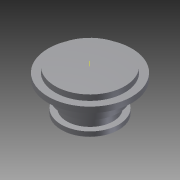
# Autodesk Inventor part: GL45 bottle cap insert; solid
Saved by Autodesk Inventor 2011 (Build 150239000, 239)
## iProperties
Created: 2012-03-14
Part Number: GL45 bottle cap insert; solid
Document SubType Name: Modeling
Designer: Marc
Density: 1 g/cm^3
Author: Marc
Autodesk Inventor part; units mm, degrees
ref_plane "YZ Plane" through (0, 0, 0) normal (1, 0, 0) x (0, 1, 0)
ref_plane "XZ Plane" through (0, 0, 0) normal (0, 1, 0) x (-1, 0, 0)
ref_plane "XY Plane" through (0, 0, 0) normal (0, 0, 1) x (1, 0, 0)
sketch "Sketch1" plane through (0, 0, 0) normal (0, 0, 1) x (1, 0, 0)
  line L0 (0, 0) -> (-14.478, 0)
  line L1 (-14.478, 0) -> (-14.478, 2.54)
  line L2 (-14.478, 2.54) -> (-11.684, 2.54)
  line L3 (-11.684, 2.54) -> (-11.684, 7.62)
  line L4 (-11.684, 7.62) -> (-14.478, 7.62)
  line L5 (-14.478, 7.62) -> (-14.478, 15.24)
  line L6 (-14.478, 15.24) -> (-21.082, 15.24)
  line L7 (-21.082, 15.24) -> (-21.082, 18.034)
  line L8 (-21.082, 18.034) -> (-17.526, 18.034)
  line L9 (-17.526, 18.034) -> (-17.526, 20.828)
  line L10 (-17.526, 20.828) -> (0, 20.828)
  line L11 (0, 20.828) -> (0, 0)
  dimension "d0" = 17.526
  dimension "d1" = 21.082
  dimension "d2" = 14.478
  dimension "d3" = 11.684
  dimension "d4" = 2.794
  dimension "d5" = 5.588
  dimension "d7" = 18.288
  dimension "d8" = 13.208
  dimension "d9" = 20.828
  constraints: 24 end point, 9 parallel, 2 collinear, 1 horizontal, 1 perpendicular
  measures "d0" distance of L9.end L10.end
  measures "d1" distance between parallel lines of L11 L7
  measures "d2" distance between parallel lines of L5 L11
  measures "d3" distance between parallel lines of L11 L3
  measures "d4" distance of L8.end L9.end
  measures "d5" distance between parallel lines of L6 L10
  measures "d7" distance between parallel lines of L2 L10
  measures "d8" distance between parallel lines of L10 L4
  measures "d9" distance between parallel lines of L0 L10
revolve "Revolution1" add sketch "Sketch1" angle 360 about axis through (0, 20.828, 0) along (0, -1, 0)
chamfer "Chamfer1" distance 0.254 angle 45 1 edges at (14.478, 0, 0)
body "Solid1"
